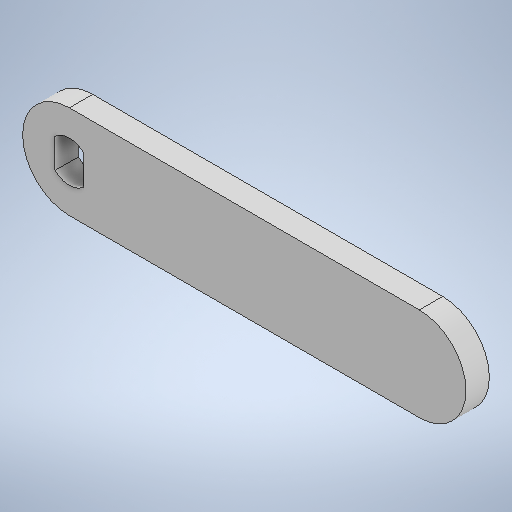
# Autodesk Inventor part: Shooting Arm V2
Saved by Autodesk Inventor 2025.4 (Build 294407000, 407)
## iProperties
Created: 2026-04-07
Part Number: Shooting Arm V2
Material: Generic
Document SubType Name: Sheet Metal
Designer: lenovo
Density: 1 g/cm^3
Sheet Metal Rule: Default_mm
Appearance: Default
Author: lenovo
Autodesk Inventor part; units mm, degrees
ref_plane "YZ Plane" through (0, 0, 0) normal (1, 0, 0) x (0, 1, 0)
ref_plane "XZ Plane" through (0, 0, 0) normal (0, 1, 0) x (-1, 0, 0)
ref_plane "XY Plane" through (0, 0, 0) normal (0, 0, 1) x (1, 0, 0)
sketch "Sketch1" plane through (0, 0, 0) normal (0, 0, 1) x (1, 0, 0)
  line L0 (0, 2.65) -> (0, -2.65)
  line L1 (-1.85, 0) -> (1.85, 0)
  line L2 (1.85, 1.8974) -> (1.85, -1.8974)
  arc A0 (1.85, 1.8974) -> (-1.85, 1.8974) centre (0, 0) ccw
  line L3 (-1.85, 1.8974) -> (-1.85, -1.8974)
  arc A1 (-1.85, -1.8974) -> (1.85, -1.8974) centre (0, 0) ccw
  line L4 (0, 0) -> (45, 0) construction
  line L5 (0, -6) -> (45, -6)
  line L6 (45, 6) -> (0, 6)
  arc A2 (0, 6) -> (0, -6) centre (0, 0) ccw
  arc A3 (45, -6) -> (45, 6) centre (45, 0) ccw
  point P0 (22.5, 0)
  dimension "d0" = 2.65
  dimension "d1" = 3.7
  dimension "d2" = 6
  dimension "d3" = 45
  measures "d0" radius of A0
  measures "d1" diameter of L2 L0
  measures "d2" radius of A2
  measures "d3" distance of L4.end L4.start
extrude "Plate1" add sketch "Sketch1" along normal blind 3
equation "\"d4\" = Thickness"
equation "\"BendRadius\" = Thickness"
equation "\"BendReliefWidth\" = Thickness"
equation "\"BendReliefDepth\" = 0.5 * Thickness"
equation "\"CornerReliefSize\" = 4 * Thickness"
equation "\"MinimumRemnant\" = 2 * Thickness"
equation "\"TransitionRadius\" = BendRadius"
equation "\"JacobiRadiusSize\" = BendRadius"
equation "\"GapSize\" = Thickness"
equation "\"Thickness\" = 3"
body "Solid1"
